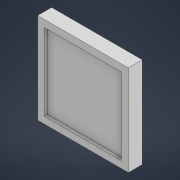
# Autodesk Inventor part: Clip_MarkerHolderV1
Saved by Autodesk Inventor 2022 (Build 260153000, 153)
## iProperties
Created: 2023-05-06
Part Number: Clip_MarkerHolderV1
Material: Generic
Document SubType Name: Modeling
Designer: Karl Spiteri
Density: 1 g/cm^3
Appearance: Default
Author: Karl Spiteri
Autodesk Inventor part; units mm, degrees
ref_plane "YZ Plane" through (0, 0, 0) normal (1, 0, 0) x (0, 1, 0)
ref_plane "XZ Plane" through (0, 0, 0) normal (0, 1, 0) x (-1, 0, 0)
ref_plane "XY Plane" through (0, 0, 0) normal (0, 0, 1) x (1, 0, 0)
sketch "Sketch1" plane through (0, 0, 0) normal (0, 0, 1) x (1, 0, 0)
  line L0 (0, 0) -> (-65, 0)
  line L1 (-65, 0) -> (-65, 65)
  line L2 (-65, 65) -> (0, 65)
  line L3 (0, 65) -> (0, 0)
  dimension "d4" = 65
  dimension "d5" = 65
  constraints: 8 end point, 2 parallel, 1 horizontal, 1 perpendicular
  measures "d4" distance of L1.end L2.end
  measures "d5" distance of L0.end L1.end
extrude "Extrusion1" add sketch "Sketch1" along normal blind 10
sketch "Sketch2" plane through (0, 0, 10) normal (0, 0, 1) x (1, 0, 0)
  line L0 (-5, 5) -> (-60, 5)
  line L1 (-60, 5) -> (-60, 60)
  line L2 (-60, 60) -> (-5, 60)
  line L3 (-5, 60) -> (-5, 5)
  point P0 (0, 0)
  dimension "d8" = 55
  dimension "d9" = 55
  constraints: 8 end point, 2 parallel, 1 horizontal, 1 perpendicular
  measures "d8" distance of L1.end L2.end
  measures "d9" distance of L0.end L1.end
extrude "Extrusion2" cut sketch "Sketch2" against normal blind 2
sketch "Sketch3" plane through (0, 0, 0) normal (0, 0, -1) x (-1, 0, 0)
  line L0 (30, 35) -> (35, 35)
  line L1 (35, 35) -> (35, 30)
  line L2 (35, 30) -> (30, 30)
  line L3 (30, 30) -> (30, 35)
  point P0 (0, 0)
  point P1 (32.5, 32.5)
  dimension "d20" = 5
  dimension "d21" = 5
  constraints: 8 end point, 2 parallel, 1 horizontal, 1 perpendicular
  measures "d20" distance of L1.end L2.end
  measures "d21" distance of L0.end L1.end
extrude "Extrusion4" cut sketch "Sketch3" against normal blind 5
body "Solid1"
